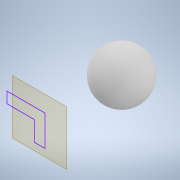
# Autodesk Inventor part: Деталь1
Saved by Autodesk Inventor 2020 (Build 240168000, 168)
## iProperties
Created: 2020-03-16
Part Number: Деталь1
Material: Типовые
Document SubType Name: Modeling
Designer: Trickster2038
Density: 1 g/cm^3
Appearance: По умолчанию
Author: Trickster2038
Autodesk Inventor part; units mm, degrees
ref_plane "YZ Plane" through (0, 0, 0) normal (1, 0, 0) x (0, 1, 0)
ref_plane "XZ Plane" through (0, 0, 0) normal (0, 1, 0) x (-1, 0, 0)
sketch "Эскиз1" plane through (0, 0, 0) normal (0, 0, 1) x (1, 0, 0)
  arc A0 (0, -35) -> (0, 35) centre (0, 0) ccw
  arc A1 (0, -45) -> (0, 45) centre (0, 0) ccw
  line L0 (0, 45) -> (0, 35)
  line L1 (0, -45) -> (0, -35)
  line L2 (0, -63) -> (0, 63) projected
  constraints: 4 end point, 4 point on circle, 2 centre point, 2 coincident, 2 point on line, 1 vertical
revolve "Вращение1" add sketch "Эскиз1" angle 360 about axis through (0, -10, 0) along (0, 1, 0) contours A0 L0 A1 L1
ref_plane "РабПлоскость1" through (0, 0, 150) normal (0, 0, 1) x (1, 0, 0)
sketch "Эскиз2" plane through (0, 0, 150) normal (0, 0, 1) x (1, 0, 0)
  line L0 (-60, 0) -> (-60, 20)
  line L1 (-60, 20) -> (10, 20)
  line L2 (10, 20) -> (10, -36)
  line L3 (-10, 0) -> (-60, 0)
  line L4 (-10, 0) -> (-10, -36)
  line L5 (-10, -36) -> (10, -36)
  point P0 (0, 0)
  constraints: 12 end point, 4 perpendicular, 1 horizontal, 1 vertical
